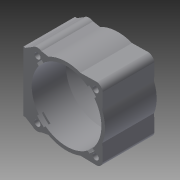
# Autodesk Inventor part: motorSupport-ExFlex-Part3
Saved by Autodesk Inventor 2014 SP2 (Build 180246200, 246)
## iProperties
Created: 2020-04-11
Part Number: motorSupport-ExFlex-Part3
Material: Generic
Document SubType Name: Sheet Metal
Designer: GauchoHP
Density: 1 g/cm^3
Sheet Metal Rule: Default_mm
Appearance: Default
Author: GauchoHP
Autodesk Inventor part; units mm, degrees
ref_plane "YZ Plane" through (0, 0, 0) normal (1, 0, 0) x (0, 1, 0)
ref_plane "XZ Plane" through (0, 0, 0) normal (0, 1, 0) x (-1, 0, 0)
ref_plane "XY Plane" through (0, 0, 0) normal (0, 0, 1) x (1, 0, 0)
sketch "Sketch2" plane through (0, 0, 0) normal (0, 1, 0) x (-1, 0, 0)
  line L0 (-12.0934, 14) -> (-15, 14)
  line L1 (-15, 14) -> (-15, 20)
  arc A0 (-13.6497, 24.4476) -> (-15, 20) centre (-7, 20) ccw
  arc A1 (13.6497, 24.4476) -> (-13.6497, 24.4476) centre (0, 0) ccw
  arc A2 (15, 20) -> (13.6497, 24.4476) centre (7, 20) ccw
  line L2 (15, 20) -> (15, 14)
  line L3 (15, 14) -> (12.0934, 14)
  arc A3 (12.0934, -14) -> (12.0934, 14) centre (0, 0) ccw
  line L4 (12.0934, -14) -> (15, -14)
  line L5 (15, -14) -> (15, -20)
  arc A4 (13.6497, -24.4476) -> (15, -20) centre (7, -20) ccw
  arc A5 (-13.6497, -24.4476) -> (13.6497, -24.4476) centre (0, 0) ccw
  arc A6 (-15, -20) -> (-13.6497, -24.4476) centre (-7, -20) ccw
  line L6 (-15, -20) -> (-15, -14)
  line L7 (-15, -14) -> (-12.0934, -14)
  arc A7 (-12.0934, 14) -> (-12.0934, -14) centre (0, 0) ccw
  line L8 (20.9594, 29.2672) -> (15.1382, 28.1928)
  arc A8 (15.1382, 28.1928) -> (-11.488, 29.8668) centre (0, 0) ccw
  line L9 (-11.488, 29.8668) -> (-25.4379, 30.1312)
  arc A9 (-25.4379, 30.1312) -> (-30.1312, 25.4379) centre (-24.25, 24.25) ccw
  line L10 (-30.1312, 25.4379) -> (-29.8668, 11.488)
  arc A10 (-29.8668, 11.488) -> (-29.8668, -11.488) centre (0, 0) ccw
  line L11 (-29.8668, -11.488) -> (-30.1312, -25.4379)
  arc A11 (-30.1312, -25.4379) -> (-25.4379, -30.1312) centre (-24.25, -24.25) ccw
  line L12 (-25.4379, -30.1312) -> (-11.488, -29.8668)
  arc A12 (-11.488, -29.8668) -> (15.1382, -28.1928) centre (0, 0) ccw
  line L13 (15.1382, -28.1928) -> (20.9594, -29.2672)
  arc A13 (20.9594, -29.2672) -> (28.4087, -28.575) centre (24.25, -24.25) ccw
  line L14 (28.4087, -28.575) -> (34.2029, -25)
  line L15 (34.2029, -25) -> (36, -25)
  line L16 (36, -25) -> (36, 25)
  line L17 (36, 25) -> (34.2029, 25)
  line L18 (34.2029, 25) -> (28.4087, 28.575)
  arc A14 (28.4087, 28.575) -> (20.9594, 29.2672) centre (24.25, 24.25) ccw
  circle A15 centre (-24.25, 24.25) radius 2
  circle A16 centre (-24.25, -24.25) radius 2
  circle A17 centre (24.25, -24.25) radius 2
  circle A18 centre (24.25, 24.25) radius 2
  circle A19 centre (0, 0) radius 18.5
  circle A20 centre (-24.25, 24.25) radius 2.5
  circle A21 centre (24.25, 24.25) radius 2.5
  circle A22 centre (-24.25, -24.25) radius 2.5
  circle A23 centre (24.25, -24.25) radius 2.5
  dimension "d12" = 5
  dimension "d13" = 5
  dimension "d14" = 5
  dimension "d15" = 5
  constraints: 38 end point, 30 point on circle, 24 centre point, 5 coincident, 1 concentric
  measures "d12" diameter of A20
  measures "d13" diameter of A21
  measures "d14" diameter of A22
  measures "d15" diameter of A23
extrude "Extrusion1" add sketch "Sketch2" along normal blind 4 contours L0 L1 A0 A1 A2 L2 L3 A19 | A19 L4 L5 A4 A5 A6 L6 L7 | A14 L18 L17 L16 L15 L14 A13 L13 A12 L12 A11 L11 A10 L10 A9 L9 A8 L8
sketch "Sketch4" plane through (0, 0, 0) normal (0, -1, 0) x (1, 0, 0)
  line L0 (-15.1382, 28.1928) -> (-20.9594, 29.2672) projected
  arc A0 (-20.9594, 29.2672) -> (-28.4087, 28.575) centre (-24.25, 24.25) ccw projected
  line L1 (-28.4087, 28.575) -> (-34.2029, 25) projected
  line L2 (-34.2029, 25) -> (-36, 25) projected
  line L3 (-36, 25) -> (-36, -25) projected
  line L4 (-36, -25) -> (-34.2029, -25) projected
  line L5 (-34.2029, -25) -> (-28.4087, -28.575) projected
  arc A1 (-28.4087, -28.575) -> (-20.9594, -29.2672) centre (-24.25, -24.25) ccw projected
  line L6 (-20.9594, -29.2672) -> (-15.1382, -28.1928) projected
  arc A2 (-15.1382, -28.1928) -> (11.488, -29.8668) centre (0, 0) ccw projected
  line L7 (11.488, -29.8668) -> (25.4379, -30.1312) projected
  arc A3 (25.4379, -30.1312) -> (30.1312, -25.4379) centre (24.25, -24.25) ccw projected
  line L8 (30.1312, -25.4379) -> (29.8668, -11.488) projected
  arc A4 (29.8668, -11.488) -> (29.8668, 11.488) centre (0, 0) ccw projected
  line L9 (29.8668, 11.488) -> (30.1312, 25.4379) projected
  arc A5 (30.1312, 25.4379) -> (25.4379, 30.1312) centre (24.25, 24.25) ccw projected
  line L10 (25.4379, 30.1312) -> (11.488, 29.8668) projected
  arc A6 (11.488, 29.8668) -> (-15.1382, 28.1928) centre (0, 0) ccw projected
  circle A7 centre (0, 0) radius 29
  circle A8 centre (-24.25, 24.25) radius 2.5 projected
  circle A9 centre (-24.25, 24.25) radius 2.5
  circle A10 centre (-24.25, -24.25) radius 2.5 projected
  circle A11 centre (24.25, -24.25) radius 2.5 projected
  circle A12 centre (24.25, 24.25) radius 2.5 projected
  circle A13 centre (24.25, 24.25) radius 2.5
  circle A14 centre (24.25, -24.25) radius 2.5
  circle A15 centre (-24.25, -24.25) radius 2.5
  dimension "d9" = 58
  dimension "d16" = 5
  dimension "d17" = 5
  constraints: 5 centre point, 5 coincident, 3 concentric
  measures "d9" diameter of A7
  measures "d16" diameter of A9
  measures "d17" diameter of A12
extrude "Extrusion2" add sketch "Sketch4" along normal blind 39
chamfer "Chamfer1" distance 10.5 angle 45 1 edges at (-29, 0, 0)
sketch "Sketch5" plane through (0, -39, 0) normal (0, -1, 0) x (1, 0, 0)
  circle A0 centre (0, 0) radius 29 projected
  arc A1 (-20.9594, 29.2672) -> (-28.4087, 28.575) centre (-24.25, 24.25) ccw projected
  arc A2 (-28.4087, -28.575) -> (-20.9594, -29.2672) centre (-24.25, -24.25) ccw projected
  arc A3 (-15.1382, -28.1928) -> (11.488, -29.8668) centre (0, 0) ccw projected
  arc A4 (25.4379, -30.1312) -> (30.1312, -25.4379) centre (24.25, -24.25) ccw projected
  arc A5 (30.1312, 25.4379) -> (25.4379, 30.1312) centre (24.25, 24.25) ccw projected
  arc A6 (11.488, 29.8668) -> (-15.1382, 28.1928) centre (0, 0) ccw projected
  line L0 (-27.8274, 31.9369) -> (37.1726, 31.9369)
  line L1 (37.1726, 31.9369) -> (37.1726, -33.0631)
  line L2 (37.1726, -33.0631) -> (-27.8274, -33.0631)
  line L3 (-27.8274, -33.0631) -> (-27.8274, 31.9369)
  circle A7 centre (0, 0) radius 27
  line L4 (0, 0) -> (-24.25, 24.25)
  line L5 (0, 0) -> (24.25, 24.25)
  line L6 (0, 0) -> (24.25, -24.25)
  line L7 (0, 0) -> (-24.25, -24.25)
  arc A8 (-18.9086, 24.5655) -> (-24.5655, 18.9086) centre (0, 0) ccw
  arc A9 (24.5655, 18.9086) -> (18.9086, 24.5655) centre (0, 0) ccw
  arc A10 (18.9086, -24.5655) -> (24.5655, -18.9086) centre (0, 0) ccw
  arc A11 (-27.8274, 13.6614) -> (-27.8274, -13.6614) centre (0, 0) ccw
  arc A12 (-24.5655, -18.9086) -> (-18.9086, -24.5655) centre (0, 0) ccw
  line L8 (-2.8284, -2.8284) -> (-21.7096, 16.0528)
  line L9 (-23.1385, 17.4817) -> (-27.0784, 21.4216)
  line L10 (2.8284, 2.8284) -> (-16.0528, 21.7096)
  line L11 (-17.4817, 23.1385) -> (-21.4216, 27.0784)
  line L12 (21.4216, 27.0784) -> (17.4817, 23.1385)
  line L13 (16.0528, 21.7096) -> (0, 5.6569)
  line L14 (27.0784, 21.4216) -> (23.1385, 17.4817)
  line L15 (21.7096, 16.0528) -> (0, -5.6569)
  line L16 (-2.8284, -2.8284) -> (16.0528, -21.7096)
  line L17 (17.4817, -23.1385) -> (21.4216, -27.0784)
  line L18 (2.8284, 2.8284) -> (21.7096, -16.0528)
  line L19 (23.1385, -17.4817) -> (27.0784, -21.4216)
  line L20 (-2.8284, 2.8284) -> (-21.7096, -16.0528)
  line L21 (-23.1385, -17.4817) -> (-27.0784, -21.4216)
  line L22 (2.8284, -2.8284) -> (-16.0528, -21.7096)
  line L23 (-17.4817, -23.1385) -> (-21.4216, -27.0784)
  line L24 (0, -5.6569) -> (-21.7096, 16.0528)
  line L25 (-23.1385, 17.4817) -> (-27.0784, 21.4216)
  line L26 (0, 5.6569) -> (-16.0528, 21.7096)
  line L27 (-17.4817, 23.1385) -> (-21.4216, 27.0784)
  dimension "d26" = 54
  dimension "d21" = 65
  dimension "d22" = 65
  dimension "d23" = 32
  dimension "d24" = 32
  constraints: 56 end point, 14 parallel, 10 point on circle, 10 point on line, 6 perpendicular, 5 centre point, 2 coincident, 1 horizontal, 19 other
  measures "d21" distance of L1.end L2.end
  measures "d22" distance of L0.end L1.end
  measures "d23" radius of A6
  measures "d24" radius of A3
extrude "Extrusion3" cut sketch "Sketch5" against normal blind 4 contours A0 L5 A9 L14 | L19 A10 L6 A0 | A0 L12 A9 L5 | L6 A10 L17 A0 | A0 L4 A8 L11 | L23 A12 L7 A0 | A0 L9 A8 L4 | L7 A12 L21 A0
equation "\"BendRadius\" = Thickness"
equation "\"BendReliefWidth\" = Thickness"
equation "\"BendReliefDepth\" = 0.5 * Thickness"
equation "\"CornerReliefSize\" = 4 * Thickness"
equation "\"MinimumRemnant\" = 2 * Thickness"
equation "\"TransitionRadius\" = BendRadius"
equation "\"JacobiRadiusSize\" = BendRadius"
equation "\"GapSize\" = Thickness"
equation "\"Thickness\" = 0.5"
body "Solid1"
